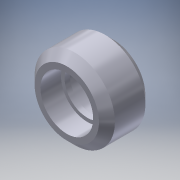
# Autodesk Inventor part: Xtreme Mini V Wheel
Saved by Autodesk Inventor 2019 (Build 230136000, 136)
## iProperties
Created: 2020-11-22
Part Number: Xtreme Mini V Wheel
Material: Rubber, Silicone
Document SubType Name: Modeling
Designer: asus
Density: 1.25 g/cm^3
Appearance: Cool White
Author: asus
Autodesk Inventor part; units mm, degrees
ref_plane "YZ Plane" through (0, 0, 0) normal (1, 0, 0) x (0, 1, 0)
ref_plane "XZ Plane" through (0, 0, 0) normal (0, 1, 0) x (-1, 0, 0)
ref_plane "XY Plane" through (0, 0, 0) normal (0, 0, 1) x (1, 0, 0)
sketch "Sketch1" plane through (0, 0, 0) normal (1, 0, 0) x (0, 1, 0)
  line L0 (-5, 0.5) -> (-4.32, 0.5)
  line L1 (-4.32, 0.5) -> (-4.32, -0.5)
  line L2 (-4.32, -0.5) -> (-5, -0.5)
  line L3 (-5, -0.5) -> (-5, -4.4)
  line L4 (-5, -4.4) -> (-6.105, -4.4)
  line L5 (-6.105, -4.4) -> (-7.615, -2.89)
  line L6 (-7.615, -2.89) -> (-7.615, 2.89)
  line L7 (-7.615, 2.89) -> (-6.105, 4.4)
  line L8 (-6.105, 4.4) -> (-5, 4.4)
  line L9 (-5, 4.4) -> (-5, 0.5)
  line L10 (0, 5.0853) -> (0, -4.725)
  point P0 (0, 0)
  point P1 (-4.32, 0)
  dimension "d0" = 2.615
  dimension "d1" = 8.8
  dimension "d2" = 5.78
  dimension "d3" = 135
  dimension "d4" = 1.105
  dimension "d6" = 1
  dimension "d7" = 0.68
  dimension "d8" = 3.9
  dimension "d9" = 10
  constraints: 22 end point, 1 horizontal alignment, 1 midpoint, 1 vertical
  measures "d0" distance between parallel lines of L3 L6
  measures "d1" distance between parallel lines of L8 L4
  measures "d2" distance of L6.start L7.start
  measures "d3" angle of L6 L5
  measures "d4" distance of L3.end L4.end
  measures "d6" distance of L0.end L1.end
  measures "d7" distance between parallel lines of L3 L1
  measures "d8" distance between parallel lines of L4 L2
  measures "d9" diameter of L9 L10
revolve "Revolution1" add sketch "Sketch1" angle 360 about axis through (0, 0, 5.0853) along (0, 0, -1)
body "Solid1"
